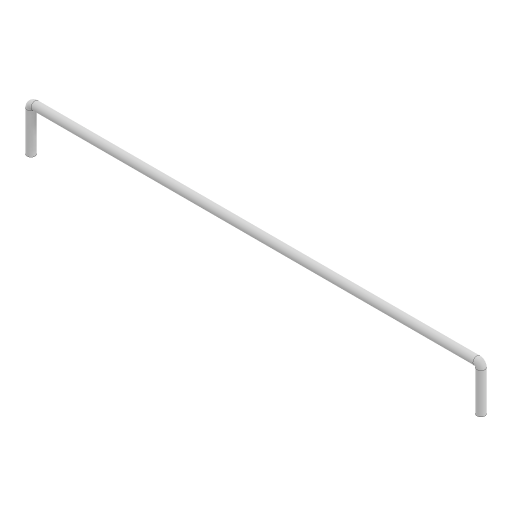
# Autodesk Inventor part: 5P.00.19.01-IB-VTP-Control-Horn
Saved by Autodesk Inventor 2024.3 (Build 283343000, 343)
## iProperties
Created: 2025-01-15
Part Number: 5P.00.19.01-IB-VTP-Control-Horn
Material: Generic
Document SubType Name: Modeling
Designer: inigo
Density: 1 g/cm^3
Appearance: Default
Author: inigo
Autodesk Inventor part; units mm, degrees
ref_plane "YZ Plane" through (0, 0, 0) normal (1, 0, 0) x (0, 1, 0)
sketch "Sketch1" plane through (0, 0, 0) normal (1, 0, 0) x (0, 1, 0)
  circle A0 centre (0, 0) radius 0.5
  dimension "d0" = 1
  constraints: 1 centre point, 1 coincident
  measures "d0" diameter of A0
extrude "Extrusion1" add sketch "Sketch1" along normal blind 54.06
ref_plane "Work Plane1" through (0, -0.5, 0) normal (0, 1, 0) x (-1, 0, 0)
sketch "Sketch2" plane through (0, -0.5, 0) normal (0, 1, 0) x (-1, 0, 0)
  circle A0 centre (-54.56, 0) radius 0.5
  line L0 (-54.06, 0.5) -> (-54.06, -0.5) projected
  point P0 (0, 0)
  dimension "d3" = 1
  dimension "d4" = 0.5
  constraints: 1 centre point
  measures "d3" diameter of A0
  measures "d4" distance from line of L0 A0.centre
sketch "Sketch3" plane through (0, 0, 0) normal (0, 0, 1) x (1, 0, 0)
  line L0 (54.06, -0.5) -> (54.06, 0.5) projected
  arc A0 (54.56, -0.5) -> (54.06, 0) centre (54.06, -0.5) ccw
  point P0 (0, 0)
  dimension "d5" = 0.5
  constraints: 2 point on circle, 1 centre point, 1 midpoint
  measures "d5" radius of A0
sweep "Sweep1" add profiles "Sketch2" path "Sketch3" path curves A0
sketch "Sketch4" plane through (54.56, -0.5, 0) normal (0, -1, 0) x (1, 0, 0)
  circle A0 centre (0, 0) radius 0.5
  point P0 (-54.56, 0)
  constraints: 1 centre point
extrude "Extrusion2" add sketch "Sketch4" along normal blind 5
ref_plane "Work Plane2" through (26.53, 0, 0) normal (-1, 0, 0) x (0, 0, 1)
mirror "Mirror1" about plane through (26.53, 0, 0) normal (-1, 0, 0)
body "Solid1"
